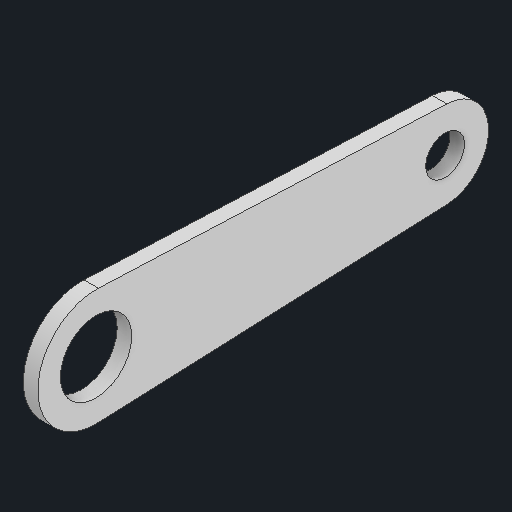
# Autodesk Inventor part: Gearbox Gusset
Saved by Autodesk Inventor 2025 (Build 290162000, 162)
## iProperties
Created: 2024-10-21
Part Number: Gearbox Gusset
Material: Generic
Document SubType Name: Modeling
Designer: Averey Ku
Density: 1 g/cm^3
Appearance: Default
Author: Averey Ku
Autodesk Inventor part; units mm, degrees
ref_plane "YZ Plane" through (0, 0, 0) normal (1, 0, 0) x (0, 1, 0)
ref_plane "XZ Plane" through (0, 0, 0) normal (0, 1, 0) x (-1, 0, 0)
ref_plane "XY Plane" through (0, 0, 0) normal (0, 0, 1) x (1, 0, 0)
sketch "Sketch1" plane through (0, 0, 0) normal (1, 0, 0) x (0, 1, 0)
  circle A0 centre (0, 0) radius 3.9
  circle A1 centre (0, -38.1) radius 2.1209
  arc A2 (6.3445, -0.2646) -> (-6.3445, -0.2646) centre (0, 0) ccw
  arc A3 (-4.7584, -38.2984) -> (4.7584, -38.2984) centre (0, -38.1) ccw
  line L0 (6.3445, -0.2646) -> (4.7584, -38.2984)
  line L1 (-6.3445, -0.2646) -> (-4.7584, -38.2984)
  dimension "d0" = 7.8
  dimension "d2" = 4.2418
  constraints: 4 centre point, 4 end point, 4 point on circle, 3 coincident, 3 tangent, 2 other
  measures "d0" diameter of A0
  measures "d2" diameter of A1
extrude "Extrusion1" add sketch "Sketch1" along normal blind 1.5875
body "Solid1"
